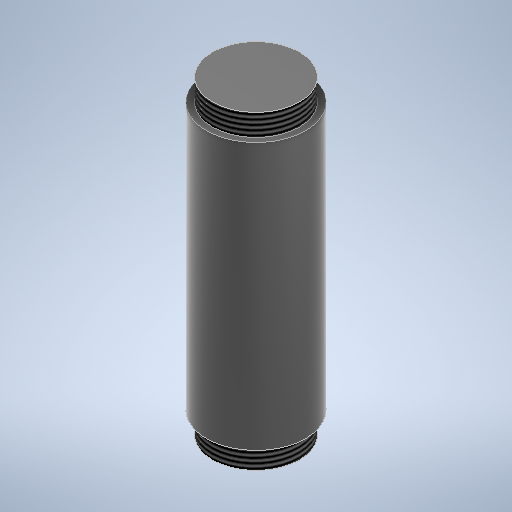
# Autodesk Inventor part: Support Tube (Filament Holder
Saved by Autodesk Inventor 2025 (Build 290162000, 162)
## iProperties
Manager: J. Wilburn
Created: 2025-03-12
Part Number: Support Tube (Filament Holder
Material: ABS Plastic
Document SubType Name: Modeling
Designer: MAL16204
Density: 1.06 g/cm^3
Appearance: Smooth - Black
Mass: 82.453 g
Surface Area: 114.857 cm^2
Volume: 77.7858 cm^3
Author: Richard Malstrom
Title: Support Tube (Filament Holder)
Subject: Ender 3 Pro Assembly
Autodesk Inventor part; units mm, degrees
ref_plane "YZ Plane" through (0, 0, 0) normal (1, 0, 0) x (0, 1, 0)
ref_plane "XZ Plane" through (0, 0, 0) normal (0, 1, 0) x (-1, 0, 0)
sketch "Sketch1" plane through (0, 0, 0) normal (0, 1, 0) x (-1, 0, 0)
  circle A0 centre (0, 0) radius 14
  dimension "d0" = 28
  constraints: 1 centre point, 1 coincident
  measures "d0" diameter of A0
extrude "Extrusion1" add sketch "Sketch1" along normal blind 100
ref_plane "Work Plane1" through (0, 7, 0) normal (0, -1, 0) x (1, 0, 0)
sketch "Sketch2" plane through (0, 7, 0) normal (0, -1, 0) x (1, 0, 0)
  circle A0 centre (0, 0) radius 16
  dimension "d4" = 32
  constraints: 1 centre point, 1 coincident
  measures "d4" diameter of A0
extrude "Extrusion2" add sketch "Sketch2" against normal blind 86
thread "Thread1" size "M30x1.5" class "6g" standard "ANSI Metric M Profile" length 7
thread "Thread2" size "M30x1.5" class "6g" standard "ANSI Metric M Profile" length 7
body "Solid1"
